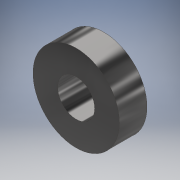
# Autodesk Inventor part: FR6ZZ Bearing_smart
Saved by Autodesk Inventor 2018 (Build 220112000, 112)
## iProperties
Created: 2015-01-19
Part Number: FR6ZZ Bearing_smart
Material: Stainless Steel
Document SubType Name: Modeling
Designer: TODD D MILLER
Mass: 19.1771 g
Surface Area: 14.9924 cm^2
Volume: 2.39714 cm^3
Density: 8 g/cm^3
Appearance: Steel - Polished
Catalog Web Link: http://www.andymark.com/product-p/am-0516.htm
Description: 3/8 in. id bearing, shielded (R6ZZ) (am-0516)
Vendor: AndyMark
Stock Number: am-0516
Author: TODD D MILLER
Autodesk Inventor part; units mm, degrees
ref_plane "YZ Plane" through (0, 0, 0) normal (1, 0, 0) x (0, 1, 0)
ref_plane "XZ Plane" through (0, 0, 0) normal (0, 1, 0) x (-1, 0, 0)
ref_plane "XY Plane" through (0, 0, 0) normal (0, 0, 1) x (1, 0, 0)
sketch "Sketch1" plane through (0, 0, 0) normal (0, 0, 1) x (1, 0, 0)
  circle A0 centre (0, 0) radius 11.1125
  dimension "d1" = 22.225
  constraints: 1 centre point, 1 coincident
  measures "d1" diameter of A0
extrude "Extrusion1" add sketch "Sketch1" against normal blind 7.112
hole "Hole1" at (0, 0, 0) direction (0, 0, -1) diameter 9.525 end through all
body "Solid2"
